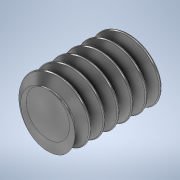
# Autodesk Inventor part: Rans10 punta plana
Saved by Autodesk Inventor 2020 (Build 240168000, 168)
## iProperties
Created: 2020-09-17
Part Number: Rans10 punta plana
Material: Steel AISI 1045 450 QT
Document SubType Name: Modeling
Designer: aaron
Density: 7.85 g/cm^3
Appearance: Steel Galvanized
Author: aaron
Autodesk Inventor part; units mm, degrees
ref_plane "YZ Plane" through (0, 0, 0) normal (1, 0, 0) x (0, 1, 0)
ref_plane "XZ Plane" through (0, 0, 0) normal (0, 1, 0) x (-1, 0, 0)
ref_plane "XY Plane" through (0, 0, 0) normal (0, 0, 1) x (1, 0, 0)
sketch "Sketch1" plane through (0, 0, 0) normal (0, 0, 1) x (1, 0, 0)
  circle A0 centre (0, 0) radius 2.413
  dimension "d0" = 4.826
  constraints: 1 centre point, 1 coincident
  measures "d0" diameter of A0
extrude "Extrusion1" add sketch "Sketch1" along normal blind 6.35
thread "Thread1" size "10-24 UNC" class "2A" standard "ANSI Unified Screw Threads" full length
fillet "Fillet1" radius 0.508 1 edges at (-2.413, 0, 6.35)
fillet "Fillet2" radius 1.016 1 edges at (-2.413, 0, 0)
sketch "Sketch2" plane through (0, 0, 0) normal (0, 0, -1) x (-1, 0, 0)
  line L0 (0.2349, -2.54) -> (-0.2349, -2.54)
  line L1 (-0.2349, -2.54) -> (-0.2349, 2.54)
  line L2 (-0.2349, 2.54) -> (0.2349, 2.54)
  line L3 (0.2349, 2.54) -> (0.2349, -2.54)
  line L4 (0.2349, -2.54) -> (-0.2349, 2.54) construction
  line L5 (-0.2349, -2.54) -> (0.2349, 2.54) construction
  point P0 (0, 0)
  dimension "d7" = 5.08
  dimension "d8" = 0.4697
  constraints: 12 end point, 2 midpoint, 2 parallel, 1 horizontal, 1 perpendicular
  measures "d7" distance of L0.end L1.end
  measures "d8" distance of L1.end L2.end
extrude "Extrusion2" cut sketch "Sketch2" against normal blind 0.762
sketch "Sketch4" plane through (0, 0, 6.35) normal (-1, 0, 0) x (0, 1, 0)
  line L0 (2.413, 0) -> (2.413, 6.35)
  line L1 (2.413, 6.35) -> (1.6283, 6.35)
  line L2 (1.6283, 6.35) -> (1.6283, 0)
  line L3 (1.6283, 0) -> (2.413, 0)
  line L4 (0, -2.6554) -> (0, 7.8537) projected
  constraints: 8 end point
revolve "Revolution1" cut sketch "Sketch4" angle 360 about axis through (0, 0, 6.35) along (0, 0, -1)
sketch "Sketch5" plane through (0, 0, 6.35) normal (-1, 0, 0) x (0, 1, 0)
  line L0 (2.413, 0) -> (2.413, 6.35)
  line L1 (2.413, 6.35) -> (1.6283, 6.35)
  line L2 (1.6283, 6.35) -> (1.6283, 0)
  line L3 (1.6283, 0) -> (2.413, 0)
  line L4 (0, -2.6554) -> (0, 7.8537) projected
  constraints: 8 end point
revolve "Revolution2" add sketch "Sketch5" angle 360 about axis through (0, 0, 6.35) along (0, 0, -1) separate body
sketch "Sketch3" plane through (0, 0, 6.35) normal (1, 0, 0) x (0, 0, -1)
  line L0 (-0.6175, -1.682) -> (-0.5293, -1.682) construction
  line L1 (0.0881, -2.3597) -> (-0.0001, -2.5291) construction
  line L2 (-1.0584, -2.5291) -> (-1.1466, -2.3597) construction
  line L3 (-0.4411, -1.682) -> (-0.5293, -1.5126) construction
  line L4 (-0.5293, -1.5126) -> (-0.6175, -1.682) construction
  line L5 (-1.0584, -2.5291) -> (-0.9702, -2.3597) construction
  line L6 (-0.4411, -1.682) -> (-0.0883, -2.3597)
  line L7 (-1.1466, -2.3597) -> (-0.9702, -2.3597) construction
  arc A0 (-1.1466, -2.3597) -> (-1.0584, -2.4132) centre (-1.0584, -2.3137) ccw construction
  line L8 (0.0881, -2.3597) -> (-0.0883, -2.3597) construction
  line L9 (-1.0584, -2.5291) -> (-1.0584, -2.3597) construction
  line L10 (-0.0001, -2.5291) -> (-0.0001, -2.3597) construction
  line L11 (-0.5293, -1.5126) -> (-0.5293, -1.6285) construction
  line L12 (-1.0584, -2.4132) -> (-0.0001, -2.4132)
  arc A1 (-1.0584, -2.4132) -> (-0.9702, -2.3597) centre (-1.0584, -2.3137) ccw
  line L13 (-0.0883, -2.3597) -> (-0.0001, -2.5291) construction
  line L14 (-0.9702, -2.3597) -> (-0.6175, -1.682)
  line L15 (-0.0001, -0.0002) -> (-0.0001, 0.0177)
  line L16 (-0.0001, 0.0177) -> (-0.0001, -0.0002)
  line L17 (-0.0001, -0.0002) -> (0.0334, -0.0002)
  arc A2 (-0.0883, -2.3597) -> (-0.0001, -2.4132) centre (-0.0001, -2.3137) ccw
  arc A3 (-0.0001, -2.4132) -> (0.0881, -2.3597) centre (-0.0001, -2.3137) ccw construction
  arc A4 (-0.5293, -1.6285) -> (-0.6175, -1.682) centre (-0.5293, -1.7279) ccw
  arc A5 (-0.4411, -1.682) -> (-0.5293, -1.6285) centre (-0.5293, -1.7279) ccw
  line L18 (-0.5293, -1.6285) -> (-0.5293, -1.682) construction
  line L19 (-0.5293, -1.682) -> (-0.4411, -1.682) construction
  dimension "d11" = 55
  dimension "d12" = 0.1694
  dimension "d13" = 0.1694
  dimension "Sketch3_ThreadOffset" = 0
  dimension "Sketch3_MajorRadius" = 2.413
  dimension "d16" = 1.0583
  dimension "Sketch3_MinorRadius" = 1.6283
  constraints: 40 end point, 12 point on circle, 10 parallel, 8 tangent, 6 centre point, 6 collinear, 2 midpoint, 2 point on line, 1 horizontal, 1 perpendicular, 3 other
  measures "d11" angle of L6 L14
  measures "d12" distance of L3.end L0.end
  measures "d13" distance of L1.end L10.end
  measures "Sketch3_ThreadOffset" distance between parallel lines of L15 L10
  measures "Sketch3_MajorRadius" distance from line of L12 L15.start
  measures "d16" distance from line of L1.end L9
  measures "Sketch3_MinorRadius" distance edge to line of A5 L17
coil "Coil1" sketch "Sketch3" operation cut axis through (0, 0, 6.35) along (0, 0, -1) pitch 1.0594 turns 7.992008 hand right bodies 2
equation "\"d11\" = d18"
equation "\"d12\" = 0.160083 * Sketch3_Pitch"
equation "\"d13\" = 0.160083 * Sketch3_Pitch"
equation "\"d16\" = Sketch3_Pitch"
equation "\"d18\" = 55deg"
equation "\"Sketch3_Pitch\" = 1.05833"
body "Solid1"
body "Solid2"
